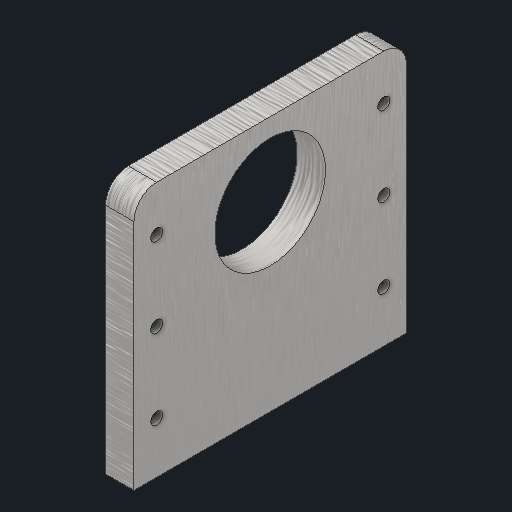
# Autodesk Inventor part: ArmSupportPlate
Saved by Autodesk Inventor 2025 (Build 290162000, 162)
## iProperties
Created: 2024-01-05
Part Number: ArmSupportPlate
Material: Aluminum 6061
Document SubType Name: Modeling
Designer: avsar
Density: 2.7 g/cm^3
Appearance: Satin Brushed
Author: avsar
Autodesk Inventor part; units mm, degrees
ref_plane "YZ Plane" through (0, 0, 0) normal (1, 0, 0) x (0, 1, 0)
ref_plane "XZ Plane" through (0, 0, 0) normal (0, 1, 0) x (-1, 0, 0)
ref_plane "XY Plane" through (0, 0, 0) normal (0, 0, 1) x (1, 0, 0)
sketch "Sketch1" plane through (0, 0, 0) normal (1, 0, 0) x (0, 1, 0)
  line L0 (-45, 48) -> (45, 48)
  line L1 (45, 48) -> (45, -48)
  line L2 (45, -48) -> (-45, -48)
  line L3 (-45, -48) -> (-45, 48)
  line L4 (-45, 48) -> (45, -48) construction
  line L5 (45, 48) -> (-45, -48) construction
  point P0 (0, 0)
  dimension "d0" = 90
  dimension "d1" = 96
  constraints: 12 end point, 2 midpoint, 2 parallel, 1 horizontal, 1 perpendicular
  measures "d0" distance of L1.end L2.end
  measures "d1" distance of L0.end L1.end
extrude "Extrusion1" add sketch "Sketch1" along normal blind 10
sketch "Sketch3" plane through (10, 0, 0) normal (1, 0, 0) x (0, 0, -1)
  circle A0 centre (0, 19) radius 19.5
  line L0 (-48, -45) -> (48, -45) projected
  point P0 (0, 0)
  point P1 (0, -45)
  dimension "d16" = 39
  dimension "d17" = 64
  constraints: 1 centre point, 1 midpoint, 1 vertical alignment
  measures "d16" diameter of A0
  measures "d17" distance of point (0, -45) A0.centre
extrude "Extrusion3" cut sketch "Sketch3" against normal through all
sketch "Sketch5" plane through (10, 0, 0) normal (1, 0, 0) x (0, 0, -1)
  circle A0 centre (-40, 29) radius 2.1
  line L0 (-48, 45) -> (-48, -45) construction
  line L1 (-48, -45) -> (48, -45) projected
  circle A1 centre (-40, 1) radius 2.1
  circle A2 centre (-40, -27) radius 2.1
  circle A3 centre (0, 19) radius 19.5 construction
  line L2 (0, 38.5) -> (0, 19) construction
  circle A4 centre (40, 29) radius 2.1
  circle A5 centre (40, 1) radius 2.1
  circle A6 centre (40, -27) radius 2.1
  point P0 (0, 0)
  point P1 (-7.5, 41)
  point P2 (7.5, 41)
  dimension "d32" = 4.2
  dimension "d33" = 8
  dimension "d34" = 74
  dimension "d37" = 28
  constraints: 6 centre point, 3 symmetric about line, 2 end point, 2 vertical, 9 other
  measures "d32" diameter of A0
  measures "d33" distance from line of L0 A0.centre
  measures "d34" distance from line of L1 A0.centre
  measures "d37" distance of A0.centre A1.centre
extrude "Extrusion5" cut sketch "Sketch5" against normal through all
sketch "Sketch6" plane through (0, -45, -48) normal (0, -1, 0) x (1, 0, 0)
  circle A0 centre (5, 90) radius 2.1
  line L0 (0, 96) -> (0, 0) construction
  line L1 (0, 96) -> (10, 96) construction
  circle A1 centre (5, 76) radius 2.1
  circle A2 centre (5, 62) radius 2.1
  circle A3 centre (5, 48) radius 2.1
  circle A4 centre (5, 34) radius 2.1
  circle A5 centre (5, 20) radius 2.1
  circle A6 centre (5, 6) radius 2.1
  point P0 (0, 48)
  point P1 (0, 48)
  point P2 (5, 96)
  dimension "d44" = 4.2
  dimension "d45" = 42
  dimension "d48" = 14
  constraints: 7 centre point, 2 midpoint, 1 vertical, 1 vertical alignment, 12 other
  measures "d44" diameter of A0
  measures "d45" vertical distance of point (0, 48) A0.centre
  measures "d48" distance of A0.centre A1.centre
extrude "Extrusion6" cut sketch "Sketch6" against normal blind 10
thread "Thread1" size "M4.5x0.75" class "6H" standard "ISO Metric profile" full length
thread "Thread2" size "M4.5x0.75" class "6H" standard "ANSI Metric M Profile" full length
thread "Thread3" size "M4.5x0.75" class "6H" standard "ANSI Metric M Profile" full length
thread "Thread4" size "M4.5x0.75" class "6H" standard "ANSI Metric M Profile" full length
thread "Thread5" size "M4.5x0.75" class "6H" standard "ANSI Metric M Profile" full length
thread "Thread6" size "M4.5x0.75" class "6H" standard "ANSI Metric M Profile" full length
thread "Thread7" size "M4.5x0.75" class "6H" standard "ANSI Metric M Profile" full length
fillet "Fillet1" radius 8 2 edges at (5, 45, 48) (5, 45, -48)
body "Solid1"
